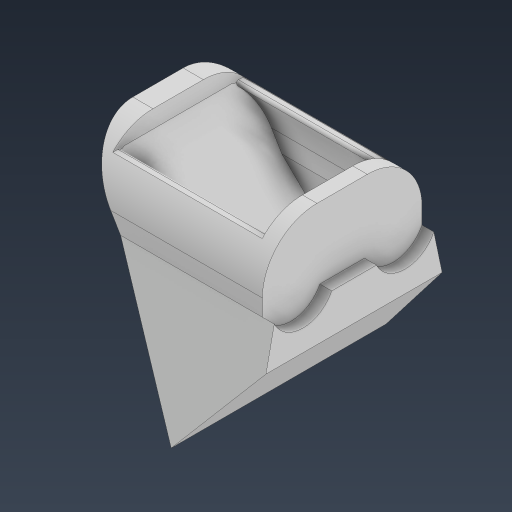
# Autodesk Inventor part: 8bitdo_Pad_stand
Saved by Autodesk Inventor 2024 (Build 280153000, 153)
## iProperties
Created: 2023-12-21
Part Number: 8bitdo_Pad_stand
Material: Generic
Document SubType Name: Modeling
Designer: Piter
Density: 1 g/cm^3
Appearance: Default
Author: Piter
Autodesk Inventor part; units mm, degrees
ref_plane "YZ Plane" through (0, 0, 0) normal (1, 0, 0) x (0, 1, 0)
ref_plane "XZ Plane" through (0, 0, 0) normal (0, 1, 0) x (-1, 0, 0)
ref_plane "XY Plane" through (0, 0, 0) normal (0, 0, 1) x (1, 0, 0)
sketch "Sketch1" plane through (0, 0, 0) normal (1, 0, 0) x (0, 1, 0)
  line L0 (10.3949, 29) -> (0.3949, 29)
  line L1 (0.3949, 29) -> (0.3949, -29)
  line L2 (0.3949, -29) -> (10.3949, -29)
  line L3 (10.3949, -29) -> (10.3949, 29)
  line L4 (10.3949, 29) -> (0.3949, -29) construction
  line L5 (0.3949, 29) -> (10.3949, -29) construction
  circle A0 centre (6.3949, 21.5) radius 13.5
  line L6 (0.3949, 29) -> (0.3949, 33.5934)
  line L7 (0.3949, 0) -> (10.3949, 0)
  line L8 (10.3949, -29) -> (0.3949, -29)
  circle A1 centre (6.3949, -21.5) radius 13.5
  line L9 (0.3949, -29) -> (0.3949, -33.5934)
  line L10 (0, 0) -> (-30, 0)
  line L11 (-30, 0) -> (-30, 40)
  line L12 (-30, 40) -> (0.3949, 33.5934)
  line L13 (0.3949, -29) -> (0.3949, -33.5934)
  line L14 (-30, 0) -> (-30, -40)
  line L15 (-30, -40) -> (0.3949, -33.5934)
  line L16 (0.3949, 33.5934) -> (30.3949, 33.5934)
  line L17 (30.3949, 33.5934) -> (30.3949, -33.5934)
  line L18 (30.3949, -33.5934) -> (0.3949, -33.5934)
  line L19 (0.3949, -33.5934) -> (0.3949, 33.5934)
  point P0 (5.3949, 0)
  point P1 (-7.1051, 21.5)
  point P2 (0.3949, 9.4066)
  point P3 (0.3949, -9.4066)
  point P4 (-7.1051, -21.5)
  dimension "d0" = 10
  dimension "d1" = 58
  dimension "d4" = 27
  dimension "d5" = 21.5
  dimension "d6" = 6
  dimension "d7" = 18.8132
  dimension "d8" = 30
  dimension "d9" = 40
  dimension "d10" = 30
  constraints: 40 end point, 7 point on circle, 6 symmetric about line, 4 midpoint, 4 parallel, 3 horizontal, 3 perpendicular, 2 centre point, 2 point on line, 1 coincident, 1 vertical, 1 other
  measures "d0" distance of L2.end L1.end
  measures "d1" distance of L1.end L0.end
  measures "d4" diameter of A0
  measures "d5" distance from line of L7 A0.centre
  measures "d6" distance from line of L1 A0.centre
  measures "d7" distance of A1.end point (0.395, 9.407)
  measures "d8" distance of L10.start L10.end
  measures "d9" distance of L10.end L11.end
  measures "d10" distance of L17.end L18.end
extrude "Extrusion1" add sketch "Sketch1" along normal blind 5 contours L3 A0 L1 L0 | L0 L6 L16 A0 L3 | L1 A0 L6 | A0 L16 L17 L18 A1 L3 | L3 L7 L1 A0 | L3 A1 L1 L7 | A1 L18 L9 L2 L3 | L3 L2 L1 A1 | L1 L9 A1
extrude "Extrusion2" add sketch "Sketch1" along normal blind 10 contours L1 A1 L15 L14 L11 L12 A0
fillet "Fillet1" radius 23 2 edges at (2.5, 30.3949, 33.5934) (2.5, 30.3949, -33.5934)
move faces "Move1" translate (-26, 0, 0) faces at (0, -19.8684, 11.1978)
sketch "Sketch2" plane through (5, 0.3949, 33.5934) normal (0, 0, 1) x (1, 0, 0)
  line L0 (5, 0) -> (5, -30.3949) projected
  line L1 (0, 30) -> (-31, 30) projected
  line L2 (5, -30.3949) -> (-31, 30)
  line L3 (-31, -30.3949) -> (5, -30.3949) projected
  line L4 (-31, 30) -> (-31, -30.3949)
  line L5 (-31, -30.3949) -> (5, -30.3949)
  point P0 (-5, -0.3949)
  constraints: 6 end point, 1 perpendicular
extrude "Extrusion3" cut sketch "Sketch2" along normal blind 12.813 and the other way blind 92.563
move faces "Move3" translate (-34.359, -20.4806, 0) faces at (3.9608, -19.8684, 11.1978)
chamfer "Chamfer2" distance 92 distance2 62 1 edges at (10, -108.1226, 0) measured on face at (10, -107.6226, 0)
sketch "Sketch4" plane through (5, 30.3949, 10.5934) normal (0, 1, 0) x (1, 0, 0)
  line L0 (-6.1329, 37.87) -> (-69.0521, 37.87)
  line L1 (-69.0521, 37.87) -> (-69.0521, -18.4261)
  line L2 (-69.0521, -18.4261) -> (-6.1329, -18.4261)
  line L3 (-6.1329, -18.4261) -> (-6.1329, 37.87)
  point P0 (-5, 10.5934)
  constraints: 8 end point, 2 parallel, 1 horizontal, 1 perpendicular
extrude "Extrusion4" cut sketch "Sketch4" against normal blind 7.437
shell "Shell1" thickness 3.25 removed faces 1 at (-22.106, 22.9579, 9.26)
fillet "Fillet2" radius 1 2 edges at (-32.5925, 22.9579, -22.753) (-32.5925, 22.9579, 22.753)
body "Solid1"
